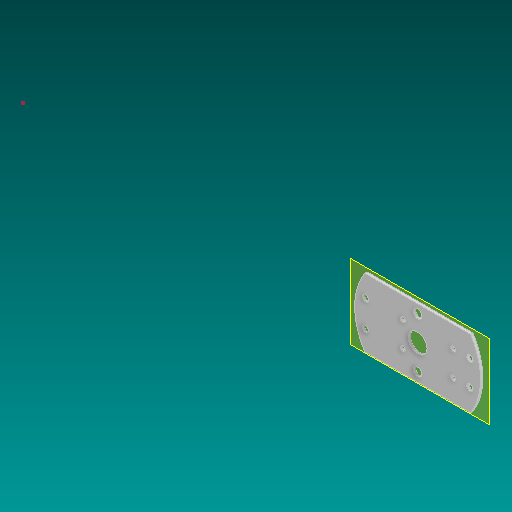
# Autodesk Inventor part: Part17
Saved by Autodesk Inventor 2020 (Build 240168000, 168)
## iProperties
Created: 2022-11-15
Part Number: Part17
Material: 一般
Document SubType Name: Modeling
Designer: Administrator
Density: 1 g/cm^3
Appearance: 既定
Author: Administrator
Autodesk Inventor part; units mm, degrees
ref_plane "YZ Plane" through (0, 0, 0) normal (1, 0, 0) x (0, 1, 0)
ref_plane "XZ Plane" through (0, 0, 0) normal (0, 1, 0) x (-1, 0, 0)
ref_plane "XY Plane" through (0, 0, 0) normal (0, 0, 1) x (1, 0, 0)
sketch "スケッチ1" plane through (0, 0, 0) normal (0, 0, 1) x (1, 0, 0)
  point P0 (0, 0)
ref_plane "作業平面1" through (242.6146, -15.2304, -10) normal (0, 0, 1) x (1, 0, 0)
sketch "スケッチ2" plane through (242.6146, -15.2304, -10) normal (0, 0, 1) x (1, 0, 0)
  line L0 (-33.6666, -21.6) -> (33.6666, -21.6) projected
  arc A0 (33.6666, -21.6) -> (33.6666, 21.6) centre (0, 0) ccw projected
  line L1 (33.6666, 21.6) -> (-33.6666, 21.6) projected
  arc A1 (-33.6666, 21.6) -> (-33.6666, -21.6) centre (0, 0) ccw projected
  circle A2 centre (33.25, -8) radius 2 projected
  circle A3 centre (33.25, 8) radius 2 projected
  circle A4 centre (22.5, 8) radius 1.6 projected
  circle A5 centre (22.5, -8) radius 1.6 projected
  line L2 (-4.9746, -0.5032) -> (-4.9749, 0.5004) projected
  arc A6 (-4.9746, -0.5032) -> (-4.9749, 0.5004) centre (0, 0) ccw projected
  circle A7 centre (-33.25, 8) radius 2 projected
  circle A8 centre (-9.5, -8) radius 1.6 projected
  circle A9 centre (-9.5, 8) radius 1.6 projected
  circle A10 centre (-33.25, -9) radius 2 projected
  circle A11 centre (0, 0) radius 6
  circle A12 centre (0, 16) radius 2.75 projected
  circle A13 centre (0, -16) radius 2.75 projected
  point P0 (-242.6146, 15.2304)
  dimension "d0" = 12
  constraints: 1 centre point, 1 coincident
  measures "d0" diameter of A11
extrude "押し出し1" add sketch "スケッチ2" along normal blind 1.5 contours A1 L1 A0 L0
